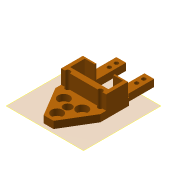
# Autodesk Inventor part: 30_Cube_Z_Focus_MGN12_NEMA_slide_part2
Saved by Autodesk Inventor 2019.4 (Build 234330000, 330)
## iProperties
Created: 2021-04-25
Part Number: 30_Cube_Z_Focus_MGN12_NEMA_slide_part2
Material: Generic
Document SubType Name: Modeling
Designer: diederichbenedict
Density: 1 g/cm^3
Appearance: Orange
Author: diederichbenedict
Autodesk Inventor part; units mm, degrees
ref_plane "YZ Plane" through (0, 0, 0) normal (1, 0, 0) x (0, 1, 0)
ref_plane "XZ Plane" through (0, 0, 0) normal (0, 1, 0) x (-1, 0, 0)
ref_plane "XY Plane" through (0, 0, 0) normal (0, 0, 1) x (1, 0, 0)
ref_plane "Work Plane8" through (-7.4556, -16.4352, 24.63) normal (0, 1, 0) x (0, 0, -1)
sketch "Sketch12" plane through (-7.4556, -16.4352, 24.63) normal (0, 1, 0) x (0, 0, -1)
  line L0 (59.1648, 4.9103) -> (72.1552, 12.4103) construction
  arc A0 (80.66, 7.5) -> (72.1552, 12.4103) centre (70.66, 0) ccw construction
  line L1 (80.66, 7.5) -> (80.66, -7.5) construction
  arc A1 (72.1552, -12.4103) -> (80.66, -7.5) centre (70.66, 0) ccw construction
  line L2 (72.1552, -12.4103) -> (59.1648, -4.9103) construction
  arc A2 (59.1648, 4.9103) -> (59.1648, -4.9103) centre (70.66, 0) ccw construction
  line L3 (57.3131, 5.945) -> (46.6951, 5.945) construction
  line L4 (46.6951, 5.945) -> (46.6951, -5.9961)
  line L5 (46.6951, -5.9961) -> (57.3131, -5.9961)
  line L6 (57.3131, -5.9961) -> (57.3131, -15)
  line L7 (57.3131, -15) -> (85.66, -15) construction
  line L8 (85.66, -15) -> (85.66, 15) construction
  line L9 (85.66, 15) -> (57.3131, 15) construction
  line L10 (57.3131, 15) -> (57.3131, 5.945) construction
  line L11 (46.6951, -6.3061) -> (57.3131, -6.3061)
  line L12 (41.63, -16.87) -> (45.71, -16.87) projected
  line L13 (55.66, -15) -> (46.2855, -13.3689) projected
  line L14 (55.66, -15) -> (105.1976, -15) construction
  line L15 (46.6951, 0) -> (46.6951, -6.3061)
  line L16 (9.71, -3.1754) -> (12.46, -1.5877) construction
  line L17 (12.46, -1.5877) -> (12.46, 1.5877) construction
  line L18 (12.46, 1.5877) -> (9.71, 3.1754) construction
  line L19 (9.71, 3.1754) -> (6.96, 1.5877) construction
  line L20 (6.96, 1.5877) -> (6.96, -1.5877) construction
  line L21 (6.96, -1.5877) -> (9.71, -3.1754) construction
  line L22 (-3.79, -3.4952) -> (-3.79, 3.4952)
  line L23 (-3.79, 0) -> (-3.79, 0)
  line L24 (-3.79, 0) -> (-3.79, -3.4952)
  line L25 (-3.79, -3.4952) -> (16.8576, -15.8838)
  line L26 (46.6951, 0) -> (-3.79, 0)
  line L27 (57.3131, -6.3061) -> (57.3131, -15)
  line L28 (57.3131, -15) -> (37.3669, -15)
  line L29 (-3.79, -8.16) -> (-3.79, 8.16) projected
  line L30 (19.46, 16.4952) -> (10.1021, 16.4952) projected
  line L31 (19.46, -16.4952) -> (19.46, 16.4952) projected
  line L32 (10.1021, -16.4952) -> (19.46, -16.4952) projected
  line L33 (10.1021, 16.4952) -> (-3.79, 8.16) projected
  line L34 (-3.79, -8.16) -> (10.1021, -16.4952) projected
  line L35 (16.8576, -15.8838) -> (37.0553, -15.8838)
  line L36 (37.0553, -15.8838) -> (37.2259, -15)
  line L37 (37.2259, -15) -> (37.3669, -15)
  line L38 (24.71, 0) -> (35.01, 0)
  line L39 (35.01, 0) -> (35.01, -13.8)
  line L40 (35.01, -13.8) -> (24.71, -13.8)
  line L41 (24.71, -13.8) -> (24.71, 0)
  line L42 (37.71, -16.97) -> (3.77, -16.97) construction
  line L43 (3.77, 16.97) -> (37.71, 16.97) projected
  arc A3 (33.3973, -5.8482) -> (33.5394, -6.05) centre (33.6783, -5.8013) ccw projected
  line L44 (33.5394, -6.05) -> (37.71, -6.05) projected
  line L45 (37.71, -6.05) -> (37.71, 6.05) projected
  line L46 (33.5394, 6.05) -> (37.71, 6.05) projected
  arc A4 (33.5394, 6.05) -> (33.3973, 5.8482) centre (33.6783, 5.8013) ccw projected
  arc A5 (33.0041, 5.5514) -> (33.3973, 5.8482) centre (32.4953, 6.6343) ccw projected
  arc A6 (33.0041, 5.5514) -> (32.8929, 5.425) centre (33.1246, 5.3332) ccw projected
  line L47 (32.8541, 4.928) -> (32.8929, 5.425) projected
  arc A7 (32.6355, 4.7) -> (32.8541, 4.928) centre (32.6056, 4.9475) ccw projected
  line L48 (32.1844, 4.7) -> (32.6355, 4.7) projected
  arc A8 (31.9361, 4.9275) -> (32.1844, 4.7) centre (32.1844, 4.9493) ccw projected
  line L49 (31.9042, 5.293) -> (31.9361, 4.9275) projected
  arc A9 (31.9042, 5.293) -> (31.7512, 5.5514) centre (31.6564, 5.3208) ccw projected
  arc A10 (31.2333, 5.8954) -> (31.7512, 5.5514) centre (32.1426, 6.7024) ccw projected
  arc A11 (31.2333, 5.8954) -> (31.01, 6.05) centre (31.0027, 5.8008) ccw projected
  line L50 (30.41, 6.05) -> (31.01, 6.05) projected
  line L51 (29.91, 5.55) -> (30.41, 6.05) projected
  line L52 (29.91, 5.55) -> (29.91, -5.55) projected
  line L53 (29.91, -5.55) -> (30.41, -6.05) projected
  line L54 (30.41, -6.05) -> (31.01, -6.05) projected
  arc A12 (31.01, -6.05) -> (31.2333, -5.8954) centre (31.0027, -5.8008) ccw projected
  arc A13 (31.7512, -5.5514) -> (31.2333, -5.8954) centre (32.1426, -6.7024) ccw projected
  arc A14 (31.7512, -5.5514) -> (31.9042, -5.293) centre (31.6564, -5.3208) ccw projected
  line L55 (31.9042, -5.293) -> (31.9361, -4.9275) projected
  arc A15 (32.1844, -4.7) -> (31.9361, -4.9275) centre (32.1844, -4.9493) ccw projected
  line L56 (32.1844, -4.7) -> (32.6355, -4.7) projected
  arc A16 (32.8541, -4.928) -> (32.6355, -4.7) centre (32.6056, -4.9475) ccw projected
  line L57 (32.8541, -4.928) -> (32.8929, -5.425) projected
  arc A17 (32.8929, -5.425) -> (33.0041, -5.5514) centre (33.1246, -5.3332) ccw projected
  arc A18 (33.3973, -5.8482) -> (33.0041, -5.5514) centre (32.4953, -6.6343) ccw projected
  arc A19 (33.3366, -5.8448) -> (32.8372, -5.2672) centre (32.2262, -6.3) ccw construction
  arc A20 (32.7155, -5.0738) -> (32.8372, -5.2672) centre (32.9645, -5.052) ccw construction
  line L58 (32.7155, -5.0738) -> (32.6853, -4.7282) construction
  arc A21 (32.6853, -4.7282) -> (32.4362, -4.5) centre (32.4362, -4.75) ccw construction
  line L59 (32.4362, -4.5) -> (31.9838, -4.5) construction
  arc A22 (31.9838, -4.5) -> (31.7347, -4.7282) centre (31.9838, -4.75) ccw construction
  line L60 (31.7347, -4.7282) -> (31.7027, -5.0948) construction
  arc A23 (31.5868, -5.2845) -> (31.7027, -5.0948) centre (31.4536, -5.073) ccw construction
  arc A24 (31.5868, -5.2845) -> (31.1159, -5.8448) centre (32.2262, -6.3) ccw construction
  arc A25 (30.8846, -6) -> (31.1159, -5.8448) centre (30.8846, -5.75) ccw construction
  line L61 (30.8846, -6) -> (30.21, -6) construction
  line L62 (30.21, -6) -> (29.71, -5.5) construction
  line L63 (29.71, -5.5) -> (29.71, 5.5) construction
  line L64 (29.71, 5.5) -> (30.21, 6) construction
  line L65 (30.21, 6) -> (30.8846, 6) construction
  arc A26 (31.1159, 5.8448) -> (30.8846, 6) centre (30.8846, 5.75) ccw construction
  arc A27 (31.1159, 5.8448) -> (31.5868, 5.2845) centre (32.2262, 6.3) ccw construction
  arc A28 (31.7027, 5.0948) -> (31.5868, 5.2845) centre (31.4536, 5.073) ccw construction
  line L66 (31.7027, 5.0948) -> (31.7347, 4.7282) construction
  arc A29 (31.7347, 4.7282) -> (31.9838, 4.5) centre (31.9838, 4.75) ccw construction
  line L67 (31.9838, 4.5) -> (32.4362, 4.5) construction
  arc A30 (32.4362, 4.5) -> (32.6853, 4.7282) centre (32.4362, 4.75) ccw construction
  line L68 (32.6853, 4.7282) -> (32.7155, 5.0738) construction
  arc A31 (32.8372, 5.2672) -> (32.7155, 5.0738) centre (32.9645, 5.052) ccw construction
  arc A32 (32.8372, 5.2672) -> (33.3366, 5.8448) centre (32.2262, 6.3) ccw construction
  arc A33 (33.5679, 6) -> (33.3366, 5.8448) centre (33.5679, 5.75) ccw construction
  line L69 (33.5679, 6) -> (34.71, 6) construction
  line L70 (34.71, 6) -> (34.71, 12.9) construction
  line L71 (34.71, 12.9) -> (34.11, 13.5) construction
  line L72 (34.11, 13.5) -> (30.71, 13.5) construction
  arc A34 (29.91, 13.5) -> (30.71, 13.5) centre (30.31, 13.8) ccw construction
  line L73 (29.91, 13.5) -> (25.31, 13.5) construction
  line L74 (25.31, 13.5) -> (24.71, 12.9) construction
  line L75 (24.71, 12.9) -> (24.71, 6.4) construction
  line L76 (24.71, 6.4) -> (25.11, 6) construction
  line L77 (25.11, 6) -> (25.11, -6) construction
  line L78 (25.11, -6) -> (24.71, -6.4) construction
  line L79 (24.71, -6.4) -> (24.71, -12.9) construction
  line L80 (24.71, -12.9) -> (25.31, -13.5) construction
  line L81 (25.31, -13.5) -> (34.11, -13.5) construction
  line L82 (34.11, -13.5) -> (34.71, -12.9) construction
  line L83 (34.71, -12.9) -> (34.71, -6) construction
  line L84 (34.71, -6) -> (33.5679, -6) construction
  arc A35 (33.3366, -5.8448) -> (33.5679, -6) centre (33.5679, -5.75) ccw construction
  point P0 (24.63, -7.4556)
  point P1 (11.21, -12.4952)
  point P2 (19.46, 12.4952)
  point P3 (19.46, -12.4952)
  dimension "d114" = 6.05
  dimension "d115" = 6.05
  dimension "d116" = 0.3
  dimension "d117" = 0.3
  constraints: 40 end point, 7 point on line, 3 horizontal, 3 parallel, 3 perpendicular, 3 vertical, 1 coincident, 1 midpoint, 2 other
  measures "d114" distance between parallel lines of L26 L44
  measures "d115" distance between parallel lines of L46 L26
  measures "d116" distance between parallel lines of L81 L40
  measures "d117" distance from line of L82.end L39
extrude "Extrusion11" add sketch "Sketch12" along normal blind 5 contours L4 L15 L11 L6 L28 L37 L36 L35 L31 L26 L41 L40 L39 L44 L45 | L5 L6 L11 L15 | L45 L44 L39 L26 | L39 L44 A3 A18 A17 L57 A16 L56 A15 L55 A14 A13 A12 L54 L53 L52 L26 | L52 L53 L54 A12 A13 A14 L55 A15 L56 A16 L57 A17 A18 A3 L44 L39 L40 L41 L26 | L31 L35 L25 L22 L26
sketch "Sketch13" plane through (-7.4556, -11.4352, 24.63) normal (0, 1, 0) x (1, 0, 0)
  line L0 (-13.1744, 24.9113) -> (13.5, 24.9113)
  line L1 (13.5, 24.9113) -> (13.5, 35.2113)
  line L2 (13.5, 35.2113) -> (-13.1744, 35.2113)
  line L3 (-13.1744, 35.2113) -> (-13.1744, 24.9113)
  line L4 (-13.5, 34.3113) -> (-13.5, 26.5113) construction
  line L5 (-13.5, 26.5113) -> (-12.3, 25.3113) construction
  line L6 (-12.3, 25.3113) -> (11.7, 25.3113) construction
  line L7 (11.7, 25.3113) -> (12.9, 26.5113) construction
  line L8 (12.9, 26.5113) -> (12.9, 34.3113) construction
  line L9 (12.9, 34.3113) -> (12.3, 34.9113) construction
  line L10 (12.3, 34.9113) -> (5.7, 34.9113) construction
  line L11 (5.7, 34.9113) -> (5.7, 33.7692) construction
  arc A0 (5.5448, 33.5379) -> (5.7, 33.7692) centre (5.45, 33.7692) ccw construction
  arc A1 (5.5448, 33.5379) -> (4.9672, 33.0386) centre (6, 32.4276) ccw construction
  arc A2 (4.7738, 32.9168) -> (4.9672, 33.0386) centre (4.752, 33.1659) ccw construction
  line L12 (4.7738, 32.9168) -> (4.4282, 32.8866) construction
  arc A3 (4.4282, 32.8866) -> (4.2, 32.6375) centre (4.45, 32.6375) ccw construction
  line L13 (4.2, 32.6375) -> (4.2, 32.1851) construction
  arc A4 (4.2, 32.1851) -> (4.4282, 31.9361) centre (4.45, 32.1851) ccw construction
  line L14 (4.4282, 31.9361) -> (4.7947, 31.904) construction
  arc A5 (4.9845, 31.7882) -> (4.7947, 31.904) centre (4.773, 31.6549) ccw construction
  arc A6 (4.9845, 31.7882) -> (5.5448, 31.3172) centre (6, 32.4276) ccw construction
  arc A7 (5.7, 31.0859) -> (5.5448, 31.3172) centre (5.45, 31.0859) ccw construction
  line L15 (5.7, 31.0859) -> (5.7, 30.4113) construction
  line L16 (5.7, 30.4113) -> (5.2, 29.9113) construction
  line L17 (5.2, 29.9113) -> (-5.8, 29.9113) construction
  line L18 (-5.8, 29.9113) -> (-6.3, 30.4113) construction
  line L19 (-6.3, 30.4113) -> (-6.3, 31.0859) construction
  arc A8 (-6.1448, 31.3172) -> (-6.3, 31.0859) centre (-6.05, 31.0859) ccw construction
  arc A9 (-6.1448, 31.3172) -> (-5.5845, 31.7882) centre (-6.6, 32.4276) ccw construction
  arc A10 (-5.3948, 31.904) -> (-5.5845, 31.7882) centre (-5.373, 31.6549) ccw construction
  line L20 (-5.3948, 31.904) -> (-5.0282, 31.9361) construction
  arc A11 (-5.0282, 31.9361) -> (-4.8, 32.1851) centre (-5.05, 32.1851) ccw construction
  line L21 (-4.8, 32.1851) -> (-4.8, 32.6375) construction
  arc A12 (-4.8, 32.6375) -> (-5.0282, 32.8866) centre (-5.05, 32.6375) ccw construction
  line L22 (-5.0282, 32.8866) -> (-5.3738, 32.9168) construction
  arc A13 (-5.5672, 33.0386) -> (-5.3738, 32.9168) centre (-5.352, 33.1659) ccw construction
  arc A14 (-5.5672, 33.0386) -> (-6.1448, 33.5379) centre (-6.6, 32.4276) ccw construction
  arc A15 (-6.3, 33.7692) -> (-6.1448, 33.5379) centre (-6.05, 33.7692) ccw construction
  line L23 (-6.3, 33.7692) -> (-6.3, 34.9113) construction
  line L24 (-6.3, 34.9113) -> (-12.9, 34.9113) construction
  line L25 (-12.9, 34.9113) -> (-13.5, 34.3113) construction
  circle A16 centre (-7.2, 27.9063) radius 2.1 construction
  circle A17 centre (6.6, 27.9063) radius 2.1 construction
  arc A18 (5.5448, 33.5379) -> (4.9672, 33.0386) centre (6, 32.4276) ccw construction
  arc A19 (4.7738, 32.9168) -> (4.9672, 33.0386) centre (4.752, 33.1659) ccw construction
  line L26 (4.7738, 32.9168) -> (4.4282, 32.8866) construction
  arc A20 (4.4282, 32.8866) -> (4.2, 32.6375) centre (4.45, 32.6375) ccw construction
  line L27 (4.2, 32.6375) -> (4.2, 32.1851) construction
  arc A21 (4.2, 32.1851) -> (4.4282, 31.9361) centre (4.45, 32.1851) ccw construction
  line L28 (4.4282, 31.9361) -> (4.7948, 31.904) construction
  arc A22 (4.9845, 31.7882) -> (4.7948, 31.904) centre (4.773, 31.6549) ccw construction
  arc A23 (4.9845, 31.7882) -> (5.5448, 31.3172) centre (6, 32.4276) ccw construction
  arc A24 (5.7, 31.0859) -> (5.5448, 31.3172) centre (5.45, 31.0859) ccw construction
  line L29 (5.7, 31.0859) -> (5.7, 30.4113) construction
  line L30 (5.7, 30.4113) -> (5.2, 29.9113) construction
  line L31 (5.2, 29.9113) -> (-5.8, 29.9113) construction
  line L32 (-5.8, 29.9113) -> (-6.3, 30.4113) construction
  line L33 (-6.3, 30.4113) -> (-6.3, 31.0859) construction
  arc A25 (-6.1448, 31.3172) -> (-6.3, 31.0859) centre (-6.05, 31.0859) ccw construction
  arc A26 (-6.1448, 31.3172) -> (-5.5846, 31.7882) centre (-6.6, 32.4276) ccw construction
  arc A27 (-5.3948, 31.904) -> (-5.5846, 31.7882) centre (-5.373, 31.6549) ccw construction
  line L34 (-5.3948, 31.904) -> (-5.0282, 31.9361) construction
  arc A28 (-5.0282, 31.9361) -> (-4.8, 32.1851) centre (-5.05, 32.1851) ccw construction
  line L35 (-4.8, 32.1851) -> (-4.8, 32.6375) construction
  arc A29 (-4.8, 32.6375) -> (-5.0282, 32.8866) centre (-5.05, 32.6375) ccw construction
  line L36 (-5.0282, 32.8866) -> (-5.3738, 32.9168) construction
  arc A30 (-5.5672, 33.0386) -> (-5.3738, 32.9168) centre (-5.3521, 33.1659) ccw construction
  arc A31 (-5.5672, 33.0386) -> (-6.1448, 33.5379) centre (-6.6, 32.4276) ccw construction
  arc A32 (-6.3, 33.7692) -> (-6.1448, 33.5379) centre (-6.05, 33.7692) ccw construction
  line L37 (-6.3, 33.7692) -> (-6.3, 34.9113) construction
  line L38 (-6.3, 34.9113) -> (-13.2, 34.9113) construction
  line L39 (-13.2, 34.9113) -> (-13.8, 34.3113) construction
  line L40 (-13.8, 34.3113) -> (-13.8, 30.9113) construction
  arc A33 (-13.8, 30.1113) -> (-13.8, 30.9113) centre (-14.1, 30.5113) ccw construction
  line L41 (-13.8, 30.1113) -> (-13.8, 25.5113) construction
  line L42 (-13.8, 25.5113) -> (-13.2, 24.9113) construction
  line L43 (-13.2, 24.9113) -> (-6.7, 24.9113) construction
  line L44 (-6.7, 24.9113) -> (-6.3, 25.3113) construction
  line L45 (-6.3, 25.3113) -> (5.7, 25.3113) construction
  line L46 (5.7, 25.3113) -> (6.1, 24.9113) construction
  line L47 (6.1, 24.9113) -> (12.6, 24.9113) construction
  line L48 (12.6, 24.9113) -> (13.2, 25.5113) construction
  line L49 (13.2, 25.5113) -> (13.2, 34.3113) construction
  line L50 (13.2, 34.3113) -> (12.6, 34.9113) construction
  line L51 (12.6, 34.9113) -> (5.7, 34.9113) construction
  line L52 (5.7, 34.9113) -> (5.7, 33.7692) construction
  arc A34 (5.5448, 33.5379) -> (5.7, 33.7692) centre (5.45, 33.7692) ccw construction
  point P0 (7.4556, 24.63)
  dimension "d110" = 0.3
  dimension "d111" = 0.3
  constraints: 8 end point, 2 parallel, 1 horizontal, 1 perpendicular, 1 point on line
  measures "d110" distance between parallel lines of L49 L1
  measures "d111" distance between parallel lines of L2 L10
extrude "Extrusion12" cut sketch "Sketch13" against normal through all
sketch "Sketch16" plane through (-7.4556, -11.4352, 24.63) normal (0, 1, 0) x (1, 0, 0)
  line L0 (5.9961, 46.6951) -> (0, 46.6951) projected
  line L1 (13.8689, 40.3869) -> (13.8689, 45.71) projected
  line L2 (15, 39.0186) -> (13.3086, 39.0186)
  line L3 (13.3086, 39.0186) -> (13.3086, 58.901)
  line L4 (13.3086, 58.901) -> (15, 58.901)
  line L5 (15, 58.901) -> (15, 39.0186)
  arc A0 (15, 37.3669) -> (13.3086, 39.0186) centre (7.8235, 31.71) ccw
  line L6 (13.3086, 58.901) -> (15, 60.5924)
  line L7 (15, 37.3669) -> (15, 57.3131) projected
  line L8 (13.3086, 58.901) -> (15.7006, 58.901) construction
  line L9 (15, 60.5924) -> (15, 58.901)
  line L10 (15, 39.0186) -> (15, 37.3669)
  line L11 (3.4952, -3.79) -> (15.8838, 16.8576) projected
  line L12 (15, 37.2259) -> (15, 57.3131) projected
  line L13 (15, 57.3131) -> (5.9961, 57.3131) projected
  line L14 (5.9961, 57.3131) -> (5.9961, 46.6951) projected
  line L15 (0, 24.9113) -> (0, -3.79) projected
  line L16 (0, -3.79) -> (3.4952, -3.79) projected
  line L17 (15.8838, 16.8576) -> (15.8838, 37.0553) projected
  line L18 (15.8838, 37.0553) -> (15, 37.2259) projected
  line L19 (13.5, 24.9113) -> (0, 24.9113) projected
  line L20 (0, 46.6951) -> (0, 35.2113) projected
  line L21 (0, 35.2113) -> (13.5, 35.2113) projected
  line L22 (13.5, 35.2113) -> (13.5, 24.9113) projected
  point P0 (7.4556, 24.63)
  dimension "d80" = 45
  constraints: 16 end point, 4 point on line, 2 horizontal, 2 parallel, 2 point on circle, 1 centre point, 1 equal length, 1 perpendicular, 1 vertical
  measures "d80" angle of L8 L6
extrude "Extrusion15" cut sketch "Sketch16" against normal through all contours L13 L5 L2 L3 | L3 L4 L5 L13 | L2 L7 A0 | L6 L9 L4
mirror "Mirror3" about plane through (-7.4556, -16.4352, -22.0651) normal (-1, 0, 0) of "Extrusion11", "Extrusion12", "Extrusion15"
sketch "Sketch17" plane through (-7.4556, -11.4352, 24.63) normal (0, 1, 0) x (1, 0, 0)
  circle A0 centre (6.4952, 13.46) radius 4 projected
  circle A1 centre (0, 2.21) radius 4 projected
  circle A2 centre (-6.4952, 13.46) radius 4 projected
  point P0 (7.4556, 24.63)
extrude "Extrusion16" cut sketch "Sketch17" against normal blind 4.5
sketch "Sketch18" plane through (-7.4556, -11.4352, 24.63) normal (0, 1, 0) x (1, 0, 0)
  line L0 (-15.8838, 37.0553) -> (-15.8838, 16.8576) projected
  line L1 (15.8838, 37.0553) -> (15.8838, 16.8576) projected
  line L2 (15.8838, 24.956) -> (15.8838, 20.956)
  line L3 (15.8838, 20.956) -> (-15.8838, 20.956)
  line L4 (-15.8838, 20.956) -> (-15.8838, 24.956)
  line L5 (15, 37.3669) -> (15, 37.2259) projected
  line L6 (-15, 37.2259) -> (15, 37.2259) construction
  line L7 (-15.8838, 36.3069) -> (15.8838, 36.3069)
  line L8 (15.8838, 16.8576) -> (15.8838, 37.0553) projected
  line L9 (-15.8838, 36.3069) -> (15.8838, 36.3069) construction
  line L10 (-13.5, 35.2113) -> (13.5, 35.2113)
  line L11 (13.5, 35.2113) -> (13.5, 24.9113)
  line L12 (13.5, 24.9113) -> (-13.5, 24.9113)
  line L13 (-13.5, 24.9113) -> (-13.5, 35.2113)
  line L14 (-15.8838, 36.3069) -> (15.8838, 36.3069)
  line L15 (15.8838, 36.3069) -> (15.8838, 20.956)
  line L16 (15.8838, 20.956) -> (-15.8838, 20.956)
  line L17 (-15.8838, 20.956) -> (-15.8838, 36.3069)
  point P0 (7.4556, 24.63)
  dimension "d85" = 4
  dimension "d96" = 0
  constraints: 28 end point, 5 parallel, 4 horizontal, 4 point on line, 2 perpendicular, 1 collinear
  measures "d85" distance of L2.start L2.end
  measures "d96" distance between parallel lines of L7 L9
extrude "Extrusion17" add sketch "Sketch18" along normal blind 10
sketch "Sketch19" plane through (-23.3393, -11.4352, 3.674) normal (0, 0, 1) x (1, 0, 0)
  circle A0 centre (5.8838, 6.8) radius 1.25 projected
  circle A1 centre (25.8838, 6.8) radius 1.25 projected
  point P0 (23.3393, 11.4352)
  point P1 (6.1474, 5.1418)
  point P2 (26.1474, 5.1418)
hole "Hole1" at (-17.4556, -4.6352, 3.674) at (2.5444, -4.6352, 3.674) direction (0, 0, -1) diameter 3.2 end through all
sketch "Sketch20" plane through (-7.4556, -11.4352, 24.63) normal (0, 1, 0) x (1, 0, 0)
  circle A0 centre (-9.5825, 53.6267) radius 1.4 projected
  circle A1 centre (9.7314, 53.6267) radius 1.4 projected
  arc A2 (-9.1809, 47.2855) -> (-9.9842, 47.2855) centre (-9.5825, 48.6267) ccw projected
  arc A3 (10.133, 47.2855) -> (9.3297, 47.2855) centre (9.7314, 48.6267) ccw projected
  circle A4 centre (-9.5825, 48.6267) radius 1.4
  circle A5 centre (9.7314, 48.6267) radius 1.4
  point P0 (7.4556, 24.63)
  constraints: 2 centre point, 2 coincident, 2 concentric
extrude "Extrusion18" cut sketch "Sketch20" against normal blind 10
sketch "Sketch21" plane through (-7.4556, -1.4352, 24.63) normal (0, 1, 0) x (1, 0, 0)
  line L0 (-13.1744, 33.91) -> (-13.1744, 26.11) projected
  line L1 (-13.1744, 26.11) -> (-11.9744, 24.91) projected
  line L2 (-11.9744, 24.91) -> (12.0256, 24.91) projected
  line L3 (12.0256, 24.91) -> (13.2256, 26.11) projected
  line L4 (13.2256, 26.11) -> (13.2256, 33.91) projected
  line L5 (13.2256, 33.91) -> (12.6256, 34.51) projected
  line L6 (12.6256, 34.51) -> (6.0256, 34.51) projected
  line L7 (6.0256, 34.51) -> (6.0256, 33.3679) projected
  arc A0 (5.8704, 33.1366) -> (6.0256, 33.3679) centre (5.7756, 33.3679) ccw projected
  arc A1 (5.8704, 33.1366) -> (5.2928, 32.6373) centre (6.3256, 32.0262) ccw projected
  arc A2 (5.0994, 32.5155) -> (5.2928, 32.6373) centre (5.0776, 32.7645) ccw projected
  line L8 (5.0994, 32.5155) -> (4.7538, 32.4853) projected
  arc A3 (4.7538, 32.4853) -> (4.5256, 32.2362) centre (4.7756, 32.2362) ccw projected
  line L9 (4.5256, 32.2362) -> (4.5256, 31.7838) projected
  arc A4 (4.5256, 31.7838) -> (4.7538, 31.5348) centre (4.7756, 31.7838) ccw projected
  line L10 (4.7538, 31.5348) -> (5.1203, 31.5027) projected
  arc A5 (5.3101, 31.3868) -> (5.1203, 31.5027) centre (5.0985, 31.2536) ccw projected
  arc A6 (5.3101, 31.3868) -> (5.8704, 30.9159) centre (6.3256, 32.0262) ccw projected
  arc A7 (6.0256, 30.6846) -> (5.8704, 30.9159) centre (5.7756, 30.6846) ccw projected
  line L11 (6.0256, 30.6846) -> (6.0256, 30.01) projected
  line L12 (6.0256, 30.01) -> (5.5256, 29.51) projected
  line L13 (5.5256, 29.51) -> (-5.4744, 29.51) projected
  line L14 (-5.4744, 29.51) -> (-5.9744, 30.01) projected
  line L15 (-5.9744, 30.01) -> (-5.9744, 30.6846) projected
  arc A8 (-5.8192, 30.9159) -> (-5.9744, 30.6846) centre (-5.7244, 30.6846) ccw projected
  arc A9 (-5.8192, 30.9159) -> (-5.259, 31.3868) centre (-6.2744, 32.0262) ccw projected
  arc A10 (-5.0692, 31.5027) -> (-5.259, 31.3868) centre (-5.0474, 31.2536) ccw projected
  line L16 (-5.0692, 31.5027) -> (-4.7026, 31.5347) projected
  arc A11 (-4.7026, 31.5347) -> (-4.4744, 31.7838) centre (-4.7244, 31.7838) ccw projected
  line L17 (-4.4744, 31.7838) -> (-4.4744, 32.2362) projected
  arc A12 (-4.4744, 32.2362) -> (-4.7026, 32.4853) centre (-4.7244, 32.2362) ccw projected
  line L18 (-4.7026, 32.4853) -> (-5.0482, 32.5155) projected
  arc A13 (-5.2416, 32.6373) -> (-5.0482, 32.5155) centre (-5.0265, 32.7645) ccw projected
  arc A14 (-5.2416, 32.6373) -> (-5.8192, 33.1366) centre (-6.2744, 32.0262) ccw projected
  arc A15 (-5.9744, 33.3679) -> (-5.8192, 33.1366) centre (-5.7244, 33.3679) ccw projected
  line L19 (-5.9744, 33.3679) -> (-5.9744, 34.51) projected
  line L20 (-5.9744, 34.51) -> (-12.5744, 34.51) projected
  line L21 (-12.5744, 34.51) -> (-13.1744, 33.91) projected
  circle A16 centre (-6.8744, 27.505) radius 2.1 projected
  circle A17 centre (6.9256, 27.505) radius 2.1 projected
  line L22 (-6.4744, 28.46) -> (6.5256, 28.46)
  line L23 (6.5256, 28.46) -> (6.5256, 59.0305)
  line L24 (6.5256, 59.0305) -> (-6.4744, 59.0305)
  line L25 (-6.4744, 59.0305) -> (-6.4744, 28.46)
  point P0 (7.4556, 24.63)
  dimension "d99" = 0.5
  dimension "d100" = 0.5
  constraints: 8 end point, 2 parallel, 1 horizontal, 1 perpendicular
  measures "d99" distance between parallel lines of L19 L25
  measures "d100" distance from line of L23 L6.end
extrude "Extrusion19" cut sketch "Sketch21" against normal through all contours L25 L24 L23 L6 L7 A0 A1 A2 L8 A3 L9 A4 L10 A5 A6 A7 L11 L12 L13 L14 L15 A8 A9 A10 L16 A11 L17 A12 L18 A13 A14 A15 L19 L20 | L20 L19 A15 A14 A13 L18 A12 L17 A11 L16 A10 A9 A8 L15 L14 L13 L12 L11 A7 A6 A5 L10 A4 L9 A3 L8 A2 A1 A0 L7 L6 L23 A17 L22 A16 L25 | A16 L22 L25 | A17 L23 L22 picked at (-5.5817, 28.592) picked at (5.6329, 28.592)
sketch "Sketch22" plane through (-7.4556, -11.4352, 24.63) normal (0, 1, 0) x (1, 0, 0)
  circle A0 centre (0, 9.71) radius 1.5 projected
  circle A1 centre (0, 9.71) radius 3
  point P0 (7.4556, 24.63)
  dimension "d103" = 6
  constraints: 1 centre point, 1 coincident
  measures "d103" diameter of A1
extrude "Extrusion20" cut sketch "Sketch22" against normal blind 10 contours A0 | A1
sketch "Sketch23" plane through (-7.4556, -11.4352, 24.63) normal (0, 1, 0) x (1, 0, 0)
  circle A0 centre (11.5, 21.21) radius 1.025 projected
  circle A1 centre (-11.5, 21.21) radius 1.25 projected
  circle A2 centre (11.5, 21.21) radius 1.75
  circle A3 centre (-11.5, 21.21) radius 1.75
  point P0 (7.4556, 24.63)
  dimension "d106" = 3.5
  dimension "d107" = 3.5
  constraints: 2 centre point, 2 coincident
  measures "d106" diameter of A2
  measures "d107" diameter of A3
extrude "Extrusion21" cut sketch "Sketch23" along normal through all both and the other way through all contours A0 | A1 | A2 | A3
body "Solid2"
